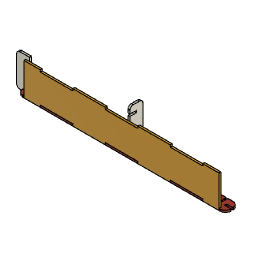
PCB Tray (Autodesk Fusion 360 design; units mm, degrees)
Autodesk Fusion 360 part; units mm, degrees
sketch "Sketch1" plane through (0, 0, 0) normal (0, 0, 1) x (1, 0, 0)
  line L0 (0, 0) -> (160, 0)
  line L1 (160, 0) -> (160, 20)
  line L2 (160, 20) -> (0, 20)
  line L3 (8.5, 28) -> (6.5, 28)
  line L4 (6.5, 28) -> (6.5, 12)
  line L5 (6.5, 12) -> (8.5, 12)
  line L6 (8.5, 12) -> (8.5, 28)
  line L7 (8.5, 28) -> (6.5, 12) construction
  line L8 (6.5, 28) -> (8.5, 12) construction
  line L9 (0, 39) -> (0, -26) construction
  line L10 (23.5, 12) -> (23.5, 28)
  line L11 (21.5, 12) -> (23.5, 12)
  line L12 (21.5, 28) -> (21.5, 12)
  line L13 (23.5, 28) -> (21.5, 28)
  line L14 (38.5, 12) -> (38.5, 28)
  line L15 (36.5, 12) -> (38.5, 12)
  line L16 (36.5, 28) -> (36.5, 12)
  line L17 (38.5, 28) -> (36.5, 28)
  line L18 (53.5, 12) -> (53.5, 28)
  line L19 (51.5, 12) -> (53.5, 12)
  line L20 (51.5, 28) -> (51.5, 12)
  line L21 (53.5, 28) -> (51.5, 28)
  line L22 (68.5, 12) -> (68.5, 28)
  line L23 (66.5, 12) -> (68.5, 12)
  line L24 (66.5, 28) -> (66.5, 12)
  line L25 (68.5, 28) -> (66.5, 28)
  line L26 (83.5, 12) -> (83.5, 28)
  line L27 (81.5, 12) -> (83.5, 12)
  line L28 (81.5, 28) -> (81.5, 12)
  line L29 (83.5, 28) -> (81.5, 28)
  line L30 (98.5, 12) -> (98.5, 28)
  line L31 (96.5, 12) -> (98.5, 12)
  line L32 (96.5, 28) -> (96.5, 12)
  line L33 (98.5, 28) -> (96.5, 28)
  line L34 (113.5, 12) -> (113.5, 28)
  line L35 (111.5, 12) -> (113.5, 12)
  line L36 (111.5, 28) -> (111.5, 12)
  line L37 (113.5, 28) -> (111.5, 28)
  line L38 (128.5, 12) -> (128.5, 28)
  line L39 (126.5, 12) -> (128.5, 12)
  line L40 (126.5, 28) -> (126.5, 12)
  line L41 (128.5, 28) -> (126.5, 28)
  line L42 (143.5, 12) -> (143.5, 28)
  line L43 (141.5, 12) -> (143.5, 12)
  line L44 (141.5, 28) -> (141.5, 12)
  line L45 (143.5, 28) -> (141.5, 28)
  line L46 (150, 8.5) -> (170, 8.5)
  line L47 (170, 8.5) -> (170, 11.5)
  line L48 (170, 11.5) -> (150, 11.5)
  line L49 (150, 11.5) -> (150, 8.5)
  line L50 (150, 8.5) -> (170, 11.5) construction
  line L51 (170, 8.5) -> (150, 11.5) construction
  line L52 (-128.5, 28) -> (-126.5, 28)
  line L53 (-141.5, 12) -> (-143.5, 12)
  line L54 (-81.5, 28) -> (-81.5, 12)
  line L55 (-111.5, 12) -> (-113.5, 12)
  line L56 (-83.5, 28) -> (-81.5, 28)
  line L57 (-126.5, 12) -> (-128.5, 12)
  line L58 (-126.5, 28) -> (-126.5, 12)
  line L59 (-111.5, 28) -> (-111.5, 12)
  line L60 (-83.5, 12) -> (-83.5, 28)
  line L61 (-170, 8.5) -> (-170, 11.5)
  line L62 (-6.5, 28) -> (-8.5, 12) construction
  line L63 (-150, 11.5) -> (-150, 8.5)
  line L64 (-81.5, 12) -> (-83.5, 12)
  line L65 (-96.5, 12) -> (-98.5, 12)
  line L66 (-150, 8.5) -> (-170, 8.5)
  line L67 (-21.5, 12) -> (-23.5, 12)
  line L68 (-98.5, 28) -> (-96.5, 28)
  line L69 (-8.5, 28) -> (-6.5, 28)
  line L70 (-38.5, 28) -> (-36.5, 28)
  line L71 (-38.5, 12) -> (-38.5, 28)
  line L72 (-170, 8.5) -> (-150, 11.5) construction
  line L73 (-36.5, 28) -> (-36.5, 12)
  line L74 (-51.5, 12) -> (-53.5, 12)
  line L75 (-98.5, 12) -> (-98.5, 28)
  line L76 (-160, 0) -> (-160, 20)
  line L77 (-96.5, 28) -> (-96.5, 12)
  line L78 (-143.5, 12) -> (-143.5, 28)
  line L79 (-170, 11.5) -> (-150, 11.5)
  line L80 (-51.5, 28) -> (-51.5, 12)
  line L81 (-66.5, 12) -> (-68.5, 12)
  line L82 (-160, 20) -> (0, 20)
  line L83 (-128.5, 12) -> (-128.5, 28)
  line L84 (-150, 8.5) -> (-170, 11.5) construction
  line L85 (-113.5, 12) -> (-113.5, 28)
  line L86 (-6.5, 12) -> (-8.5, 12)
  line L87 (0, 0) -> (-160, 0)
  line L88 (-8.5, 12) -> (-8.5, 28)
  line L89 (-141.5, 28) -> (-141.5, 12)
  line L90 (-23.5, 12) -> (-23.5, 28)
  line L91 (-143.5, 28) -> (-141.5, 28)
  line L92 (-36.5, 12) -> (-38.5, 12)
  line L93 (-53.5, 12) -> (-53.5, 28)
  line L94 (-68.5, 12) -> (-68.5, 28)
  line L95 (-6.5, 28) -> (-6.5, 12)
  line L96 (-23.5, 28) -> (-21.5, 28)
  line L97 (-66.5, 28) -> (-66.5, 12)
  line L98 (-53.5, 28) -> (-51.5, 28)
  line L99 (-68.5, 28) -> (-66.5, 28)
  line L100 (-8.5, 28) -> (-6.5, 12) construction
  line L101 (-113.5, 28) -> (-111.5, 28)
  line L102 (-21.5, 28) -> (-21.5, 12)
  point P0 (7.5, 20)
  point P1 (160, 10)
  point P2 (-7.5, 20)
  point P3 (-160, 10)
  dimension "d1" = 20
  dimension "d2" = 160
  dimension "d3" = 2
  dimension "d4" = 16
  dimension "d5" = 7.5
  dimension "d8" = 15
  dimension "d9" = 0
  dimension "d10" = 20
  dimension "d11" = 3
  constraint coincident L0.start L87.start
  constraint horizontal L0
  constraint perpendicular L0 L1
  constraint perpendicular L1 L2
  constraint horizontal L3
  constraint perpendicular L3 L4
  constraint parallel L3 L5
  constraint parallel L4 L6
  constraint coincident L7 P0
  constraint coincident L8 P0
  constraint coincident L2 P0
  constraint vertical L9
  constraint horizontal L46
  constraint perpendicular L46 L47
  constraint parallel L46 L48
  constraint parallel L47 L49
  constraint coincident L50 P1
  constraint coincident L51 P1
  constraint midpoint L1 P1
  constraint symmetric L0.start L9 L87.start
  constraint symmetric L0.end L9 L76.start
  constraint symmetric L1.end L9 L76.end
  constraint symmetric L2.end L9 L82.end
  constraint symmetric L3.start L9 L69.start
  constraint symmetric L3.end L9 L62.start
  constraint symmetric L4.end L9 L86.start
  constraint symmetric L5.end L9 L62.end
  constraint symmetric P0 L9 P2
  constraint symmetric L9 L10.start L67.end
  constraint symmetric L9 L10.end L90.end
  constraint symmetric L9 L11.start L67.start
  constraint symmetric L9 L12.start L96.end
  constraint symmetric L9 L14.start L71.start
  constraint symmetric L9 L14.end L70.start
  constraint symmetric L9 L15.start L73.end
  constraint symmetric L9 L16.start L70.end
  constraint symmetric L9 L18.start L74.end
  constraint symmetric L9 L18.end L93.end
  constraint symmetric L9 L19.start L74.start
  constraint symmetric L9 L20.start L80.start
  constraint symmetric L9 L22.start L81.end
  constraint symmetric L9 L22.end L94.end
  constraint symmetric L9 L23.start L81.start
  constraint symmetric L9 L24.start L97.start
  constraint symmetric L9 L26.start L60.start
  constraint symmetric L9 L26.end L56.start
  constraint symmetric L9 L27.start L54.end
  constraint symmetric L9 L28.start L54.start
  constraint symmetric L9 L30.start L65.end
  constraint symmetric L9 L30.end L68.start
  constraint symmetric L9 L31.start L65.start
  constraint symmetric L9 L32.start L68.end
  constraint symmetric L9 L34.start L55.end
  constraint symmetric L9 L34.end L85.end
  constraint symmetric L9 L35.start L55.start
  constraint symmetric L9 L36.start L59.start
  constraint symmetric L9 L38.start L57.end
  constraint symmetric L9 L38.end L52.start
  constraint symmetric L9 L39.start L57.start
  constraint symmetric L9 L40.start L52.end
  constraint symmetric L9 L42.start L53.end
  constraint symmetric L9 L42.end L78.end
  constraint symmetric L9 L43.start L53.start
  constraint symmetric L9 L44.start L89.start
  constraint symmetric L9 L46.start L63.end
  constraint symmetric L9 L46.end L61.start
  constraint symmetric L9 L47.end L61.end
  constraint symmetric L9 L48.end L63.start
  constraint symmetric L9 P1 P3
  measures "d1" distance of L0.end L1.end
  measures "d2" distance of L0.start L0.end
  measures "d3" distance of L4.end L5.end
  measures "d4" distance of L3.end L4.end
  measures "d5" distance of P0 L9
  measures "d10" distance of L47.end L48.end
  measures "d11" distance of L46.end L47.end
extrude "Extrude1" add sketch "Sketch1" along normal blind 3 contours L0 L1 L2 L4 L5 L6 L10 L11 L12 L14 L15 L16 L18 L19 L20 L22 L23 L24 L26 L27 L28 L30 L31 L32 L34 L35 L36 L38 L39 L40 L42 L43 L44 L46 L48 L49 L53 L54 L55 L57 L58 L59 L60 L63 L64 L65 L66 L67 L71 L73 L74 L75 L76 L77 L78 L79 L80 L81 L82 L83 L85 L86 L87 L88 L89 L90 L92 L93 L94 L95 L97 L102 makes body 1
fillet "Fillet1" radius 1 40 edges at (-143.5, 20, 1.5) (-141.5, 20, 1.5) (-128.5, 20, 1.5) (-126.5, 20, 1.5) (-113.5, 20, 1.5) (-111.5, 20, 1.5) (-98.5, 20, 1.5) (-96.5, 20, 1.5) (-83.5, 20, 1.5) (-81.5, 20, 1.5) (-68.5, 20, 1.5) (-66.5, 20, 1.5) (-53.5, 20, 1.5) (-51.5, 20, 1.5) (-38.5, 20, 1.5) (-36.5, 20, 1.5) (-23.5, 20, 1.5) (-21.5, 20, 1.5) (-8.5, 20, 1.5) (-6.5, 20, 1.5) (6.5, 20, 1.5) (8.5, 20, 1.5) (21.5, 20, 1.5) (23.5, 20, 1.5) (36.5, 20, 1.5) (38.5, 20, 1.5) (51.5, 20, 1.5) (53.5, 20, 1.5) (66.5, 20, 1.5) (68.5, 20, 1.5) (81.5, 20, 1.5) (83.5, 20, 1.5) (96.5, 20, 1.5) (98.5, 20, 1.5) (111.5, 20, 1.5) (113.5, 20, 1.5) (126.5, 20, 1.5) (128.5, 20, 1.5) (141.5, 20, 1.5) (143.5, 20, 1.5) on bodies 1
fillet "Fillet2" radius 8 4 edges at (160, 20, 1.5) (160, 0, 1.5) (-160, 20, 1.5) (-160, 0, 1.5) on bodies 1
move_body "Move1" bodies 1 to x (1, 0, 0) y (0, 1, 0) z (0, 0, 1) at (0, 0, -25)
sketch "Sketch2" plane through (0, 0, 0) normal (0, 1, 0) x (1, 0, 0)
  line L0 (-150, 25) -> (150, 25)
  line L1 (150, 25) -> (150, -25)
  line L2 (150, -25) -> (-150, -25)
  line L3 (-150, -25) -> (-150, 25)
  line L4 (-150, 25) -> (150, -25) construction
  line L5 (150, 25) -> (-150, -25) construction
  line L6 (125, -25) -> (75, -25)
  line L7 (75, -25) -> (75, -22)
  line L8 (75, -22) -> (125, -22)
  line L9 (125, -22) -> (125, -25)
  line L10 (-125, -25) -> (-75, -25)
  line L11 (-75, -25) -> (-75, -22)
  line L12 (-75, -22) -> (-125, -22)
  line L13 (-125, -22) -> (-125, -25)
  line L14 (125, 25) -> (75, 25)
  line L15 (75, 25) -> (75, 22)
  line L16 (75, 22) -> (125, 22)
  line L17 (125, 22) -> (125, 25)
  line L18 (-125, 25) -> (-75, 25)
  line L19 (-75, 25) -> (-75, 22)
  line L20 (-75, 22) -> (-125, 22)
  line L21 (-125, 22) -> (-125, 25)
  line L22 (25, -25) -> (-25, -25)
  line L23 (-25, -25) -> (-25, -22)
  line L24 (-25, -22) -> (25, -22)
  line L25 (25, -22) -> (25, -25)
  line L26 (25, 25) -> (-25, 25)
  line L27 (-25, 25) -> (-25, 22)
  line L28 (-25, 22) -> (25, 22)
  line L29 (25, 22) -> (25, 25)
  dimension "d16" = 50
  dimension "d17" = 3
  dimension "d18" = 50
  dimension "d19" = 3
  dimension "d20" = 50
  dimension "d21" = 3
  dimension "d22" = 50
  dimension "d23" = 3
  dimension "d24" = 50
  dimension "d25" = 3
  dimension "d26" = 50
  dimension "d27" = 3
  dimension "d36" = 50
  dimension "d38" = 300
  constraint horizontal L0
  constraint perpendicular L0 L1
  constraint parallel L0 L2
  constraint parallel L1 L3
  constraint coincident L4 origin
  constraint coincident L5 origin
  constraint horizontal L6
  constraint vertical L7
  constraint horizontal L8
  constraint vertical L9
  constraint coincident L2 L6.start
  constraint horizontal L10
  constraint vertical L11
  constraint horizontal L12
  constraint vertical L13
  constraint coincident L2 L10.start
  constraint horizontal L14
  constraint vertical L15
  constraint horizontal L16
  constraint vertical L17
  constraint coincident L0 L14.start
  constraint horizontal L18
  constraint vertical L19
  constraint horizontal L20
  constraint vertical L21
  constraint coincident L0 L18.start
  constraint horizontal L22
  constraint vertical L23
  constraint horizontal L24
  constraint vertical L25
  constraint coincident L2 L22.start
  constraint horizontal L26
  constraint vertical L27
  constraint horizontal L28
  constraint vertical L29
  constraint coincident L0 L26.start
  measures "d16" distance of L6.start L6.end
  measures "d17" distance of L6.start L8.end
  measures "d18" distance of L10.start L10.end
  measures "d19" distance of L10.start L12.end
  measures "d20" distance of L14.start L14.end
  measures "d21" distance of L14.start L16.end
  measures "d22" distance of L18.start L18.end
  measures "d23" distance of L18.start L20.end
  measures "d24" distance of L22.start L22.end
  measures "d25" distance of L22.start L24.end
  measures "d26" distance of L26.start L26.end
  measures "d27" distance of L26.start L28.end
  measures "d36" distance of L0.end L1.end
  measures "d38" distance of L1.end L2.end
extrude "Extrude2" add sketch "Sketch2" along normal blind 3 separate body contours L0 L1 L2 L3 L7 L8 L9 L11 L12 L13 L15 L16 L17 L19 L20 L21 L23 L24 L25 L27 L28 L29 makes body 2
combine "Combine1" operation cut target body 1 tool bodies 2 keep tools
copy_body "CopyPasteBodies1" bodies 1 makes body 3
move_body "Move2" bodies 3 to x (1, 0, 0) y (0, 1, 0) z (0, 0, 1) at (0, 0, 47)
sketch "Sketch3" plane through (0, 8.5, 0) normal (0, 1, 0) x (-1, 0, 0)
  line L0 (150, -25) -> (160, -25)
  line L1 (160, -25) -> (160, -22)
  line L2 (160, -22) -> (150, -22)
  line L3 (150, -22) -> (150, -25)
  line L4 (150, -25) -> (170, -25)
  line L5 (170, -25) -> (170, 25)
  line L6 (170, 25) -> (150, 25)
  line L7 (150, 25) -> (150, -25)
  dimension "d37" = 50
  constraint horizontal L4
  constraint vertical L5
  constraint horizontal L6
  constraint vertical L7
  constraint coincident L0.start L3.end
  measures "d37" distance of L4.end L5.end
extrude "Extrude3" add sketch "Sketch3" along normal blind 3 separate body makes body 4
fillet "Fillet3" radius 5 2 edges at (-170, 10, -25) (-170, 10, 25) on bodies 4
copy_body "CopyPasteBodies2" bodies 4 makes body 5
move_body "Move3" bodies 5 to x (-1, 0, 0) y (0, -1, 0) z (0, 0, 1) at (0, 20, 0)
sketch "Sketch4" plane through (0, 0, 0) normal (1, 0, 0) x (0, 1, 0)
  line L0 (10, -35) -> (30, -35)
  line L1 (30, -35) -> (30, 35)
  line L2 (30, 35) -> (10, 35)
  line L3 (10, 35) -> (10, -35)
  line L4 (10, -35) -> (30, 35) construction
  line L5 (30, -35) -> (10, 35) construction
  line L6 (20, -25) -> (10, -25)
  line L7 (10, -25) -> (10, -22)
  line L8 (10, -22) -> (20, -22)
  line L9 (20, -22) -> (20, -25)
  line L10 (20, 25) -> (10, 25)
  line L11 (10, 25) -> (10, 22)
  line L12 (10, 22) -> (20, 22)
  line L13 (20, 22) -> (20, 25)
  point P0 (20, 0)
  dimension "d39" = 70
  dimension "d40" = 20
  dimension "d41" = 10
  dimension "d42" = 3
  dimension "d43" = 3
  dimension "d44" = 10
  constraint horizontal L0
  constraint perpendicular L0 L1
  constraint parallel L0 L2
  constraint parallel L1 L3
  constraint coincident L4 P0
  constraint coincident L5 P0
  constraint horizontal L6
  constraint vertical L7
  constraint horizontal L8
  constraint vertical L9
  constraint coincident L3 L7.end
  constraint horizontal L10
  constraint vertical L11
  constraint horizontal L12
  constraint vertical L13
  constraint coincident L3 L11.end
  measures "d39" distance of L0.end L1.end
  measures "d40" distance of L1.end L2.end
  measures "d41" distance of L0 L6
  measures "d42" distance of L6.start L8.end
  measures "d43" distance of L10.start L12.end
  measures "d44" distance of L2 L10
extrude "Extrude4" add sketch "Sketch4" along normal blind 3 separate body contours L0 L1 L2 L3 L6 L8 L9 L10 L12 L13 makes body 6
fillet "Fillet4" radius 5 4 edges at (1.5, 10, -35) (1.5, 30, -35) (1.5, 30, 35) (1.5, 10, 35) on bodies 6
hidden bodies 3 5
equation "d3 = SlotWidth"
equation "d11 = MaterialThickness"
equation "d12 = MaterialThickness"
equation "d17 = MaterialThickness"
equation "d19 = MaterialThickness"
equation "d21 = MaterialThickness"
equation "d23 = MaterialThickness"
equation "d25 = MaterialThickness"
equation "d27 = MaterialThickness"
equation "d28 = MaterialThickness"
equation "d30 = MaterialThickness"
equation "MaterialThickness = 3 mm" comment "Thickness of material"
equation "SlotWidth = 2 mm" comment "Slots for PCBs"
equation "TrayWidth = 50 mm"
equation "d36 = TrayWidth"
equation "d37 = TrayWidth"
equation "d39 = TrayWidth + 20 mm"
equation "d42 = MaterialThickness"
equation "d43 = MaterialThickness"
equation "d45 = MaterialThickness"
named bodies: "Side", "Base", "Side 2", "Handle", "Handle 2", "AssemblyJig"
